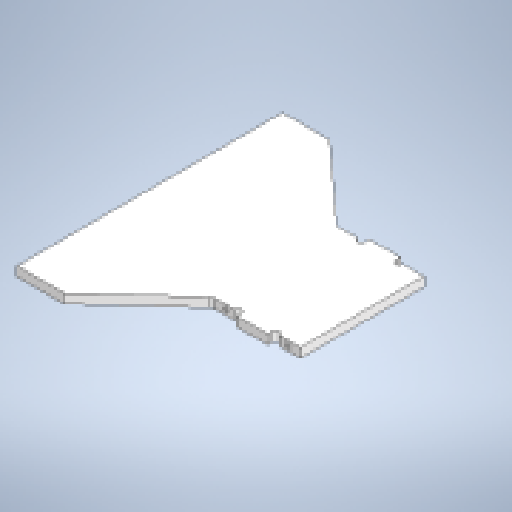
# Autodesk Inventor part: heraporika
Saved by Autodesk Inventor 2024 (Build 280153000, 153)
## iProperties
Created: 2023-12-16
Part Number: heraporika
Material: ABS プラスチック
Document SubType Name: Modeling
Designer: right
Density: 1.06 g/cm^3
Appearance: クリア
Mass: 13.5821 g
Surface Area: 194.516 cm^2
Volume: 12.8133 cm^3
Author: right
Autodesk Inventor part; units mm, degrees
ref_plane "YZ Plane" through (0, 0, 0) normal (1, 0, 0) x (0, 1, 0)
ref_plane "XZ Plane" through (0, 0, 0) normal (0, 1, 0) x (-1, 0, 0)
sketch "スケッチ1" plane through (0, 0, 0) normal (0, 0, 1) x (1, 0, 0)
  line L0 (-5.596, 10.7676) -> (-11.196, 10.7676) projected
  line L1 (-22.396, 7.7676) -> (5.604, 7.7676)
  line L2 (5.604, 7.7676) -> (5.604, 10.7676)
  line L3 (5.604, 10.7676) -> (-22.396, 10.7676)
  line L4 (-22.396, 10.7676) -> (-22.396, 7.7676)
  line L5 (-20.396, 8.7347) -> (-20.396, 10.7676) projected
  point P0 (0, 0)
  point P1 (-8.396, 10.7676)
  point P2 (-8.396, 10.7676)
  point P3 (-20.396, 9.7511)
  point P4 (-22.396, 9.2676)
  point P5 (-5.2, 11.25)
  point P6 (-10.8, 11.25)
  dimension "d0" = 3
  dimension "d1" = 2
  constraints: 8 end point, 4 midpoint, 2 parallel, 1 coincident, 1 horizontal, 1 horizontal alignment, 1 perpendicular
  measures "d0" distance of L3.end L1.start
  measures "d1" horizontal distance of point (-20.396, 9.751) point (-22.396, 9.268)
ref_plane "作業平面1" through (-20, -13.25, 39.5) normal (0, 0, -1) x (0, 1, 0)
extrude "押し出し1" add sketch "スケッチ1" along normal up to surface (39.5 mm away)
sketch "スケッチ2" plane through (-22.396, 7.7676, 0) normal (0, -1, 0) x (1, 0, 0)
  line L0 (0, 39.5) -> (28, 39.5) projected
  line L1 (9, 39.5) -> (19, 39.5)
  line L2 (19, 39.5) -> (19, 41)
  line L3 (19, 41) -> (9, 41)
  line L4 (9, 41) -> (9, 39.5)
  circle A0 centre (7.9, 39.5) radius 1.1
  line L5 (14, 41) -> (14, 39.5) construction
  line L6 (0, 0) -> (0, 39.5) construction
  line L7 (0, 19.75) -> (28, 19.75) construction
  circle A1 centre (20.1, 39.5) radius 1.1
  line L8 (9, 0) -> (19, 0)
  line L9 (19, 0) -> (19, -1.5)
  line L10 (19, -1.5) -> (9, -1.5)
  line L11 (9, -1.5) -> (9, 0)
  circle A2 centre (7.9, 0) radius 1.1
  line L12 (14, -1.5) -> (14, 0) construction
  circle A3 centre (20.1, 0) radius 1.1
  point P0 (22.396, 0)
  dimension "d6" = 2.2
  dimension "d4" = 10
  dimension "d5" = 1.5
  constraints: 22 end point, 9 symmetric about line, 3 horizontal, 3 midpoint, 2 centre point, 2 horizontal alignment, 2 parallel, 2 point on line, 1 perpendicular, 1 vertical, 1 vertical alignment, 6 other
  measures "d4" distance of L3.end L2.end
  measures "d5" distance of L2.end L1.end
extrude "押し出し2" add sketch "スケッチ2" against normal blind 3 contours L4 L3 L2 L0 | L8 L9 L10 L11
extrude "押し出し3" cut sketch "スケッチ2" against normal blind 3 contours A0 L0 | A1 L0 | L0 A1 | L0 A0 | A3 | A2
sketch "スケッチ3" plane through (-22.396, 7.7676, 39.5) normal (0, 0, 1) x (1, 0, 0)
  circle A0 centre (4, 1.5) radius 1.1 projected
  circle A1 centre (24, 1.5) radius 1.1 projected
  point P0 (22.396, -7.7676)
  constraints: 2 coincident
hole "穴1" at (-18.396, 9.2676, 39.5) at (1.604, 9.2676, 39.5) direction (0, 0, -1) diameter 1.567 end through all thread size "M2x0.4" class "6H" standard "ISO Metric profile"
sketch "スケッチ4" plane through (-22.396, 7.7676, 0) normal (0, -1, 0) x (1, 0, 0)
  line L0 (0, 0) -> (0, 39.5) projected
  line L1 (0, 39.5) -> (-42, 69.75)
  line L2 (-42, 69.75) -> (-82, 69.75)
  line L3 (-82, 69.75) -> (-82, -30.25)
  line L4 (-82, -30.25) -> (-42, -30.25)
  line L5 (6.8, 0) -> (0, 0) projected
  line L6 (-42, -30.25) -> (0, 0)
  line L7 (0, 19.75) -> (28.8198, 19.75) construction
  point P0 (22.396, 0)
  point P1 (-82, 19.75)
  dimension "d18" = 100
  dimension "d19" = 82
  dimension "d20" = 40
  constraints: 12 end point, 3 midpoint, 3 perpendicular, 1 horizontal, 1 horizontal alignment, 2 other
  measures "d18" distance between parallel lines of L4 L2
  measures "d19" distance between parallel lines of L0 L3
  measures "d20" distance of L1.end L2.end
extrude "押し出し4" add sketch "スケッチ4" against normal blind 3
fillet "フィレット1" radius 2 2 edges at (-22.396, 9.2676, 0) (-22.396, 9.2676, 39.5)
sketch "スケッチ5" plane through (5.604, 7.7676, 0) normal (0, -1, 0) x (1, 0, 0)
  arc A0 (-9, 39.5) -> (-6.8, 39.5) centre (-7.9, 39.5) ccw projected
  line L0 (-9, 39.5) -> (-9, 41) projected
  line L1 (-9, 41) -> (-19, 41) projected
  line L2 (-19, 41) -> (-19, 39.5) projected
  arc A1 (-21.2, 39.5) -> (-19, 39.5) centre (-20.1, 39.5) ccw projected
  line L3 (-27.3547, 39.5) -> (-21.2, 39.5) projected
  arc A2 (-28.5236, 39.8771) -> (-27.3547, 39.5) centre (-27.3547, 41.5) ccw projected
  line L4 (-28.5236, 39.8771) -> (-70, 69.75) projected
  line L5 (-70, 69.75) -> (-110, 69.75) projected
  line L6 (-110, 69.75) -> (-110, -30.25) projected
  line L7 (-110, -30.25) -> (-70, -30.25) projected
  line L8 (-70, -30.25) -> (-28.5236, -0.3771) projected
  arc A3 (-27.3547, 0) -> (-28.5236, -0.3771) centre (-27.3547, -2) ccw projected
  line L9 (-27.3547, 0) -> (-21.2, 0) projected
  arc A4 (-19, 0) -> (-21.2, 0) centre (-20.1, 0) ccw projected
  line L10 (-19, 0) -> (-19, -1.5) projected
  line L11 (-19, -1.5) -> (-9, -1.5) projected
  line L12 (-9, -1.5) -> (-9, 0) projected
  arc A5 (-6.8, 0) -> (-9, 0) centre (-7.9, 0) ccw projected
  line L13 (-6.8, 0) -> (0, 0) projected
  line L14 (0, 0) -> (0, 39.5) projected
  line L15 (-6.8, 39.5) -> (0, 39.5) projected
  line L16 (-70.9679, -27.25) -> (-28.9679, 3)
  line L17 (-70.9679, -27.25) -> (-107, -27.25)
  line L18 (-107, -27.25) -> (-107, 66.75)
  line L19 (-107, 66.75) -> (-70.9679, 66.75)
  line L20 (-70.9679, 66.75) -> (-28.9679, 36.5)
  line L21 (-28.9679, 36.5) -> (-3, 36.5)
  line L22 (-4.7835, 0) -> (-4.7835, 39.5) projected
  line L23 (-3, 36.5) -> (-3, 3)
  line L24 (-3.2165, 0) -> (-3.2165, 39.5) projected
  line L25 (-3, 3) -> (-28.9679, 3)
  line L26 (-70, -30.25) -> (-28.5236, -0.3771) projected
  line L27 (-110, -30.25) -> (-70, -30.25) projected
  line L28 (-110, 69.75) -> (-110, -30.25) projected
  line L29 (-70, 69.75) -> (-110, 69.75) projected
  line L30 (-28.5236, 39.8771) -> (-70, 69.75) projected
  line L31 (-27.3547, 39.5) -> (-21.2, 39.5) projected
  line L32 (-27.3547, 0) -> (-21.2, 0) projected
  line L33 (0, 0) -> (0, 39.5) projected
  line L34 (-110, -30.25) -> (-110, 69.75) construction
  line L35 (-110, 19.75) -> (-27.2262, 19.75) construction
  line L36 (-28.9679, 3) -> (-28.9679, 36.5)
  line L37 (-25.9679, 3) -> (-25.9679, 36.5)
  line L38 (-107, 19.75) -> (-28.9679, 36.5) construction
  line L39 (-107, 66.75) -> (-67.984, 28.125) construction
  line L40 (-106.2965, 67.4607) -> (-67.2804, 28.8357)
  line L41 (-67.2804, 28.8357) -> (-68.6875, 27.4143)
  line L42 (-68.6875, 27.4143) -> (-107.7035, 66.0393)
  line L43 (-107.7035, 66.0393) -> (-106.2965, 67.4607)
  line L44 (-106.2965, 67.4607) -> (-68.6875, 27.4143) construction
  line L45 (-67.2804, 28.8357) -> (-107.7035, 66.0393) construction
  line L46 (-28.5482, 35.5673) -> (-107, 18.7272)
  line L47 (-107, 18.7272) -> (-107.4197, 20.6827)
  line L48 (-107.4197, 20.6827) -> (-28.9679, 37.5228)
  line L49 (-28.9679, 37.5228) -> (-28.5482, 35.5673)
  line L50 (-28.5482, 35.5673) -> (-107.4197, 20.6827) construction
  line L51 (-107, 18.7272) -> (-28.9679, 37.5228) construction
  line L52 (-106.2965, -27.9607) -> (-67.2804, 10.6643)
  line L53 (-67.2804, 10.6643) -> (-68.6875, 12.0857)
  line L54 (-68.6875, 12.0857) -> (-107.7035, -26.5393)
  line L55 (-28.5482, 3.9327) -> (-107, 20.7728)
  line L56 (-107, 20.7728) -> (-107.4197, 18.8173)
  line L57 (-107.4197, 18.8173) -> (-28.9679, 1.9772)
  line L58 (-25.9679, 18.75) -> (-107, 18.75)
  line L59 (-107, 18.75) -> (-107, 20.75)
  line L60 (-107, 20.75) -> (-25.9679, 20.75)
  line L61 (-25.9679, 20.75) -> (-25.9679, 18.75)
  line L62 (-25.9679, 18.75) -> (-107, 20.75) construction
  line L63 (-107, 18.75) -> (-25.9679, 20.75) construction
  line L64 (-25.9679, 3) -> (-3, 36.5) construction
  line L65 (-3, 3) -> (-25.9679, 36.5) construction
  line L66 (-1.7319, 3.8031) -> (-24.7617, 37.3933)
  line L67 (-24.7617, 37.3933) -> (-27.236, 35.6969)
  line L68 (-27.236, 35.6969) -> (-4.2062, 2.1067)
  line L69 (-4.2062, 2.1067) -> (-1.7319, 3.8031)
  line L70 (-1.7319, 3.8031) -> (-27.236, 35.6969) construction
  line L71 (-24.7617, 37.3933) -> (-4.2062, 2.1067) construction
  line L72 (-1.7319, 35.6969) -> (-24.7617, 2.1067)
  line L73 (-24.7617, 2.1067) -> (-27.236, 3.8031)
  line L74 (-27.236, 3.8031) -> (-4.2062, 37.3933)
  line L75 (-4.2062, 37.3933) -> (-1.7319, 35.6969)
  line L76 (-1.7319, 35.6969) -> (-27.236, 3.8031) construction
  line L77 (-24.7617, 2.1067) -> (-4.2062, 37.3933) construction
  point P0 (-5.604, 0)
  point P1 (-88.984, 66.75)
  point P2 (-24.2774, 39.5)
  point P3 (-87.492, 47.4375)
  point P4 (-107.2099, 19.7049)
  point P5 (-67.984, 11.375)
  point P6 (-87.492, -7.9375)
  point P7 (-107.2099, 19.7951)
  point P8 (-66.484, 19.75)
  point P9 (-14.484, 19.75)
  point P10 (-14.484, 19.75)
  point P11 (-14.484, 22.4027)
  point P12 (-4.8187, 36.5)
  point P13 (-24.1492, 36.5)
  point P14 (-4.7835, 31.246)
  point P15 (-12.6653, 19.75)
  point P16 (-4.7835, 8.254)
  point P17 (-14.484, 17.0973)
  point P18 (-24.1492, 3)
  point P19 (-4.8187, 3)
  point P20 (-25.9679, 5.6527)
  point P21 (-16.3026, 19.75)
  point P22 (-25.9679, 33.8473)
  point P23 (-30.0619, 2.2121)
  point P24 (-67.6649, 10.2837)
  point P25 (-105.5786, -27.25)
  point P26 (-70.0011, 10.7852)
  point P27 (-107, 18.7272)
  point P28 (-107, -25.8429)
  point P29 (-28.9679, 20.75)
  point P30 (-28.9679, 18.75)
  point P31 (-97.5766, 20.75)
  point P32 (-28.9679, 35.4772)
  point P33 (-97.5766, 18.75)
  point P34 (-28.9679, 4.0228)
  point P35 (-107, 20.7728)
  point P36 (-70.0011, 28.7148)
  point P37 (-107, 65.3429)
  point P38 (-67.6649, 29.2163)
  point P39 (-30.0619, 37.2879)
  point P40 (-105.5786, 66.75)
  point P41 (-107, 20.7728)
  point P42 (-107, 20.7728)
  point P43 (-28.7484, 36.5)
  point P44 (-102.2352, 19.75)
  point P45 (-4.7835, 36.5513)
  point P46 (-4.7835, 36.5)
  point P47 (-25.9679, 19.75)
  dimension "d24" = 3
  dimension "d25" = 3
  dimension "d26" = 3
  dimension "d27" = 3
  dimension "d28" = 3
  dimension "d29" = 3
  dimension "d30" = 2
  dimension "d31" = 2
  dimension "d32" = 2
  dimension "d33" = 3
  dimension "d34" = 3
  constraints: 102 end point, 23 midpoint, 23 parallel, 11 symmetric about line, 10 perpendicular, 6 point on line, 2 horizontal, 1 vertical, 3 other
  measures "d24" distance between parallel lines of L18 L6
  measures "d25" distance from line of L5 point (-88.984, 66.75)
  measures "d26" distance between parallel lines of L4 L20
  measures "d27" distance from line of point (-24.277, 39.5) L21
  measures "d28" distance between parallel lines of L14 L23
  measures "d29" distance between parallel lines of L36 L37
  measures "d30" distance of L40.end L41.end
  measures "d31" distance of L46.end L47.end
  measures "d32" distance between parallel lines of L58 L60
  measures "d33" distance of L67.end L66.end
  measures "d34" distance of L72.end L73.end
extrude "押し出し5" cut sketch "スケッチ5" against normal blind 2 contours L22 L21 L74 | L74 L66 L21 | L22 L66 L72 | L74 L37 L68 | L68 L25 L72 | L60 L46 L36 | L36 L55 L58 | L48 L40 L19 L20 | L16 L17 L52 L57 | L48 L18 L42 | L57 L54 L18
sketch "スケッチ6" plane through (5.604, 9.7676, 0) normal (0, -1, 0) x (1, 0, 0)
  line L0 (-25.9679, 33.8473) -> (-16.3026, 19.75) projected
  line L1 (-16.3026, 19.75) -> (-25.9679, 5.6527) projected
  line L2 (-24.6032, 31.8569) -> (-24.6032, 7.6431) projected
  line L3 (-25.9679, 5.6527) -> (-25.9679, 33.8473) projected
  point P0 (-5.604, 0)
  point P1 (-24.6032, 36.5)
  point P2 (-24.6032, 3)
extrude "押し出し6" add sketch "スケッチ6" against normal up to surface (1 mm away)
fillet "フィレット2" radius 2 20 edges at (-101.396, 8.7676, 65.3429) (-99.9746, 8.7676, 66.75) (-65.3639, 8.7676, 66.75) (-24.4579, 8.7676, 37.2879) (-62.0609, 8.7676, 29.2163) (-64.3971, 8.7676, 28.7148) (-101.396, 8.7676, 20.7728) (-91.9726, 8.7676, 20.75) (-91.9726, 8.7676, 18.75) (-101.396, 8.7676, 18.7272) (-64.3971, 8.7676, 10.7852) (-62.0609, 8.7676, 10.2837) (-101.396, 8.7676, -25.8429) (-99.9746, 8.7676, -27.25) (-65.3639, 8.7676, -27.25) (-24.4579, 8.7676, 2.2121) (-23.3639, 8.7676, 4.0228) (-23.3639, 8.7676, 18.75) (-23.3639, 8.7676, 20.75) (-23.3639, 8.7676, 35.4772)
sketch "スケッチ9" plane through (5.604, 7.7676, 0) normal (0, -1, 0) x (1, 0, 0)
  line L0 (-107, 23.2476) -> (-107, 60.5486) projected
  arc A0 (-103.5929, 61.9699) -> (-107, 60.5486) centre (-105, 60.5486) ccw projected
  line L1 (-103.5929, 61.9699) -> (-72.6283, 31.3157) projected
  arc A1 (-73.6156, 27.9389) -> (-72.6283, 31.3157) centre (-74.0354, 29.8944) ccw projected
  line L2 (-73.6156, 27.9389) -> (-104.5803, 21.2922) projected
  arc A2 (-107, 23.2476) -> (-104.5803, 21.2922) centre (-105, 23.2476) ccw projected
  line L3 (-4.7835, 31.246) -> (-4.7835, 8.254) projected
  line L4 (-4.7835, 8.254) -> (-12.6653, 19.75) projected
  line L5 (-12.6653, 19.75) -> (-4.7835, 31.246) projected
  line L6 (-14.484, 17.0973) -> (-4.8187, 3) projected
  line L7 (-4.8187, 3) -> (-24.1492, 3) projected
  line L8 (-24.1492, 3) -> (-14.484, 17.0973) projected
  line L9 (-14.484, 22.4027) -> (-24.1492, 36.5) projected
  line L10 (-24.1492, 36.5) -> (-4.8187, 36.5) projected
  line L11 (-4.8187, 36.5) -> (-4.7835, 36.5513) projected
  line L12 (-4.7835, 36.5513) -> (-4.7835, 36.5) projected
  line L13 (-4.7835, 36.5) -> (-4.8187, 36.5) projected
  line L14 (-4.8187, 36.5) -> (-14.484, 22.4027) projected
  line L15 (-100.7156, 66.75) -> (-71.6132, 66.75) projected
  arc A3 (-70.4443, 66.3729) -> (-71.6132, 66.75) centre (-71.6132, 64.75) ccw projected
  line L16 (-70.4443, 66.3729) -> (-33.7174, 39.9208) projected
  arc A4 (-34.4666, 36.3425) -> (-33.7174, 39.9208) centre (-34.8863, 38.2979) ccw projected
  line L17 (-34.4666, 36.3425) -> (-66.607, 29.4434) projected
  arc A5 (-68.4338, 29.9775) -> (-66.607, 29.4434) centre (-67.0267, 31.3988) ccw projected
  line L18 (-68.4338, 29.9775) -> (-102.1227, 63.3287) projected
  arc A6 (-100.7156, 66.75) -> (-102.1227, 63.3287) centre (-100.7156, 64.75) ccw projected
  line L19 (-71.6132, -27.25) -> (-100.7156, -27.25) projected
  arc A7 (-102.1227, -23.8287) -> (-100.7156, -27.25) centre (-100.7156, -25.25) ccw projected
  line L20 (-102.1227, -23.8287) -> (-68.4338, 9.5225) projected
  arc A8 (-66.607, 10.0566) -> (-68.4338, 9.5225) centre (-67.0267, 8.1012) ccw projected
  line L21 (-66.607, 10.0566) -> (-34.4666, 3.1575) projected
  arc A9 (-33.7174, -0.4208) -> (-34.4666, 3.1575) centre (-34.8863, 1.2021) ccw projected
  line L22 (-33.7174, -0.4208) -> (-70.4443, -26.8729) projected
  arc A10 (-71.6132, -27.25) -> (-70.4443, -26.8729) centre (-71.6132, -25.25) ccw projected
  line L23 (-28.9679, 16.75) -> (-28.9679, 6.4976) projected
  arc A11 (-31.3876, 4.5422) -> (-28.9679, 6.4976) centre (-30.9679, 6.4976) ccw projected
  line L24 (-31.3876, 4.5422) -> (-79.1496, 14.7945) projected
  arc A12 (-78.7298, 18.75) -> (-79.1496, 14.7945) centre (-78.7298, 16.75) ccw projected
  line L25 (-78.7298, 18.75) -> (-30.9679, 18.75) projected
  arc A13 (-28.9679, 16.75) -> (-30.9679, 18.75) centre (-30.9679, 16.75) ccw projected
  line L26 (-25.9679, 5.6527) -> (-25.9679, 33.8473) projected
  line L27 (-25.9679, 33.8473) -> (-16.3026, 19.75) projected
  line L28 (-16.3026, 19.75) -> (-25.9679, 5.6527) projected
  line L29 (-79.1496, 24.7055) -> (-31.3876, 34.9578) projected
  arc A14 (-28.9679, 33.0024) -> (-31.3876, 34.9578) centre (-30.9679, 33.0024) ccw projected
  line L30 (-28.9679, 33.0024) -> (-28.9679, 22.75) projected
  arc A15 (-30.9679, 20.75) -> (-28.9679, 22.75) centre (-30.9679, 22.75) ccw projected
  line L31 (-30.9679, 20.75) -> (-78.7298, 20.75) projected
  arc A16 (-79.1496, 24.7055) -> (-78.7298, 20.75) centre (-78.7298, 22.75) ccw projected
  line L32 (-72.6283, 8.1843) -> (-103.5929, -22.4699) projected
  arc A17 (-107, -21.0486) -> (-103.5929, -22.4699) centre (-105, -21.0486) ccw projected
  line L33 (-107, -21.0486) -> (-107, 16.2524) projected
  arc A18 (-104.5803, 18.2078) -> (-107, 16.2524) centre (-105, 16.2524) ccw projected
  line L34 (-104.5803, 18.2078) -> (-73.6156, 11.5611) projected
  arc A19 (-72.6283, 8.1843) -> (-73.6156, 11.5611) centre (-74.0354, 9.6056) ccw projected
  arc A20 (-9, 39.5) -> (-6.8, 39.5) centre (-7.9, 39.5) ccw projected
  line L35 (-9, 39.5) -> (-9, 41) projected
  line L36 (-9, 41) -> (-19, 41) projected
  line L37 (-19, 41) -> (-19, 39.5) projected
  arc A21 (-21.2, 39.5) -> (-19, 39.5) centre (-20.1, 39.5) ccw projected
  line L38 (-27.3547, 39.5) -> (-21.2, 39.5) projected
  arc A22 (-28.5236, 39.8771) -> (-27.3547, 39.5) centre (-27.3547, 41.5) ccw projected
  line L39 (-28.5236, 39.8771) -> (-70, 69.75) projected
  line L40 (-70, 69.75) -> (-110, 69.75) projected
  line L41 (-110, 69.75) -> (-110, -30.25) projected
  line L42 (-110, -30.25) -> (-70, -30.25) projected
  line L43 (-70, -30.25) -> (-28.5236, -0.3771) projected
  arc A23 (-27.3547, 0) -> (-28.5236, -0.3771) centre (-27.3547, -2) ccw projected
  line L44 (-27.3547, 0) -> (-21.2, 0) projected
  arc A24 (-19, 0) -> (-21.2, 0) centre (-20.1, 0) ccw projected
  line L45 (-19, 0) -> (-19, -1.5) projected
  line L46 (-19, -1.5) -> (-9, -1.5) projected
  line L47 (-9, -1.5) -> (-9, 0) projected
  arc A25 (-6.8, 0) -> (-9, 0) centre (-7.9, 0) ccw projected
  line L48 (-6.8, 0) -> (0, 0) projected
  line L49 (0, 0) -> (0, 39.5) projected
  line L50 (-6.8, 39.5) -> (0, 39.5) projected
  line L51 (-24.1492, 36.5) -> (-25.9679, 36.5)
  line L52 (-25.9679, 36.5) -> (-25.9679, 33.8473)
  line L53 (-27.3547, 39.5) -> (-27.3547, 0)
  point P0 (-5.604, 0)
  constraints: 6 end point, 1 horizontal, 1 perpendicular, 1 vertical
extrude "押し出し9" add sketch "スケッチ9" against normal up to surface (2 mm away) contours A20 L50 L49 L48 A25 L47 L46 L45 A24 L44 L53 L38 A21 L37 L36 L35
sketch "スケッチ10" plane through (5.604, 7.7676, 0) normal (0, -1, 0) x (1, 0, 0)
  line L0 (-23.3968, 3) -> (-23.3968, 4.0975) projected
  line L1 (-4.8187, 3) -> (-23.3968, 3) projected
  line L2 (-14.484, 17.0973) -> (-4.8187, 3) projected
  line L3 (-23.3968, 4.0975) -> (-14.484, 17.0973) projected
  line L4 (-4.7835, 8.254) -> (-12.6653, 19.75) projected
  line L5 (-4.7835, 31.246) -> (-4.7835, 8.254) projected
  line L6 (-12.6653, 19.75) -> (-4.7835, 31.246) projected
  line L7 (-23.3968, 35.4025) -> (-23.3968, 36.5) projected
  line L8 (-14.484, 22.4027) -> (-23.3968, 35.4025) projected
  line L9 (-4.8187, 36.5) -> (-14.484, 22.4027) projected
  line L10 (-23.3968, 36.5) -> (-4.8187, 36.5) projected
  line L11 (-25.9679, 33.8473) -> (-16.3026, 19.75) projected
  line L12 (-25.9679, 5.6527) -> (-25.9679, 33.8473) projected
  line L13 (-16.3026, 19.75) -> (-25.9679, 5.6527) projected
  arc A0 (-22.3184, 28.5243) -> (-25.9679, 27.3933) centre (-23.9679, 27.3933) ccw
  line L14 (-14.484, 19.75) -> (-14.484, 22.4027) construction
  line L15 (-14.484, 19.75) -> (-16.3026, 19.75) construction
  arc A1 (-25.9679, 12.1067) -> (-22.3184, 10.9757) centre (-23.9679, 12.1067) ccw
  arc A2 (-22.0026, 6.1309) -> (-20.3531, 3) centre (-20.3531, 5) ccw
  line L16 (-24.1492, 3) -> (-14.484, 17.0973) construction
  line L17 (-4.8187, 3) -> (-24.1492, 3) construction
  arc A3 (-8.6148, 3) -> (-6.9653, 6.1309) centre (-8.6148, 5) ccw
  arc A4 (-20.3531, 36.5) -> (-22.0026, 33.3691) centre (-20.3531, 34.5) ccw
  arc A5 (-6.9653, 33.3691) -> (-8.6148, 36.5) centre (-8.6148, 34.5) ccw
  arc A6 (-11.8899, 20.8809) -> (-11.8899, 18.6191) centre (-10.2403, 19.75) ccw
  line L18 (-12.6653, 19.75) -> (-4.7835, 31.246) construction
  line L19 (-4.7835, 8.254) -> (-12.6653, 19.75) construction
  arc A7 (-4.7835, 24.792) -> (-8.433, 25.9229) centre (-6.7835, 24.792) ccw
  line L20 (-4.7835, 31.246) -> (-4.7835, 8.254) construction
  arc A8 (-8.433, 13.5771) -> (-4.7835, 14.708) centre (-6.7835, 14.708) ccw
  line L21 (-24.1492, 36.5) -> (-4.8187, 36.5) projected
  line L22 (-14.484, 22.4027) -> (-24.1492, 36.5) projected
  line L23 (-22.0026, 6.1309) -> (-24.1492, 3)
  line L24 (-20.3531, 3) -> (-24.1492, 3)
  point P0 (-5.604, 0)
  point P1 (-22.3184, 10.9757)
  point P2 (-25.9679, 12.1067)
  point P3 (-20.3531, 3)
  point P4 (-22.0026, 6.1309)
  point P5 (-6.9653, 6.1309)
  point P6 (-8.6148, 3)
  point P7 (-4.7835, 14.708)
  point P8 (-8.6148, 36.5)
  point P9 (-6.9653, 33.3691)
  point P10 (-22.0026, 33.3691)
  point P11 (-23.3968, 4.0975)
  dimension "d52" = 2
  dimension "d53" = 2
  dimension "d54" = 2
  dimension "d55" = 2
  constraints: 18 point on circle, 15 symmetric about line, 10 tangent, 9 centre point, 8 end point, 8 point on line, 1 collinear, 1 perpendicular, 1 vertical, 5 other
  measures "d52" radius of A0
  measures "d53" radius of A2
  measures "d54" radius of A6
  measures "d55" radius of A7
extrude "押し出し10" add sketch "スケッチ10" against normal up to surface (2 mm away) contours L24 L23 L0 | L0 L3 A2 L1 | A3 L2 L1 | L4 A8 L5 | L4 L6 A6 | A7 L6 L5 | L22 L21 L7 | L7 L10 A4 L8 | L10 L9 A5 | L11 A0 L12 | A1 L13 L12
sketch "スケッチ11" plane through (5.604, 9.7676, 0) normal (0, -1, 0) x (1, 0, 0)
  line L0 (-44.7, 39.5) -> (-44.7, 41) projected
  line L1 (-44.7, 39.5) -> (-21.7049, 39.5) projected
  line L2 (-21.7049, 41) -> (-21.7049, 39.5) projected
  line L3 (-44.7, 41) -> (-21.7049, 41) projected
  line L4 (-44.7, -1.5) -> (-44.7, 0) projected
  line L5 (-44.7, -1.5) -> (-21.7049, -1.5) projected
  line L6 (-21.7049, 0) -> (-21.7049, -1.5) projected
  line L7 (-44.7, 0) -> (-21.7049, 0) projected
  line L8 (-33.7174, -0.4208) -> (-70.4443, -26.8729) projected
  line L9 (-70.4443, 66.3729) -> (-33.7174, 39.9208) projected
  arc A0 (-34.4666, 36.3425) -> (-33.7174, 39.9208) centre (-34.8863, 38.2979) ccw projected
  arc A1 (-33.7174, -0.4208) -> (-34.4666, 3.1575) centre (-34.8863, 1.2021) ccw projected
  point P0 (-5.604, 0)
  point P1 (-33.2879, 39.5)
  point P2 (-35.2158, 41)
  point P3 (-35.2158, -1.5)
  point P4 (-33.2879, 0)
extrude "押し出し11" add sketch "スケッチ11" along normal up to surface (2 mm away) contours L0 L3 L9 A0 L1 | L4 L7 A1 L8 L5
fillet "フィレット4" radius 2 4 edges at (-29.6118, 8.7676, 41) (-27.6839, 8.7676, 39.5) (-29.6118, 8.7676, -1.5) (-27.6839, 8.7676, 0)
equation "\"d27\" = d26"
